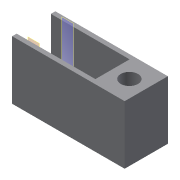
# Autodesk Inventor part: XRailVerticalExtension
Saved by Autodesk Inventor 2018 (Build 220112000, 112)
## iProperties
Created: 2019-02-14
Part Number: XRailVerticalExtension
Material: Generic
Document SubType Name: Modeling
Designer: ball
Density: 1 g/cm^3
Appearance: Default
Author: ball
Autodesk Inventor part; units mm, degrees
ref_plane "YZ Plane" through (0, 0, 0) normal (1, 0, 0) x (0, 1, 0)
ref_plane "XZ Plane" through (0, 0, 0) normal (0, 1, 0) x (-1, 0, 0)
ref_plane "XY Plane" through (0, 0, 0) normal (0, 0, 1) x (1, 0, 0)
ref_plane "Work Plane1" through (0, 0, 0) normal (0, 0, 1) x (1, 0, 0)
sketch "Sketch1" plane through (0, 0, 0) normal (0, 0, 1) x (1, 0, 0)
  line L0 (3, 16.51) -> (-3, 16.51) construction
  line L1 (-3, -16.51) -> (3, -16.51) construction
  line L2 (-9.525, -16.51) -> (-9.525, 173.99) construction
  line L3 (9.525, -16.51) -> (9.525, 173.99) construction
  line L4 (-9.525, -16.51) -> (53.975, -16.51)
  line L5 (53.975, -16.51) -> (53.975, 16.51)
  line L6 (53.975, 16.51) -> (-9.525, 16.51)
  line L7 (-9.525, 16.51) -> (-9.525, -16.51)
  point P0 (0, 0)
  dimension "d0" = 63.5
  constraints: 8 end point, 2 parallel, 1 horizontal, 1 perpendicular
  measures "d0" distance of L6.end L5.end
extrude "Extrusion1" add sketch "Sketch1" along normal blind 2.54
ref_plane "Work Plane2" through (0, 0, -19.304) normal (0, 0, -1) x (1, 0, 0)
sketch "Sketch2" plane through (0, 0, -19.304) normal (0, 0, -1) x (1, 0, 0)
  line L0 (-9.525, 16.51) -> (53.975, 16.51) projected
  line L1 (53.975, -16.51) -> (-9.525, -16.51) projected
  line L2 (-9.525, 16.51) -> (53.975, 16.51)
  line L3 (53.975, 16.51) -> (53.975, -16.51)
  line L4 (53.975, -16.51) -> (-9.525, -16.51)
  line L5 (-9.525, -16.51) -> (-9.525, 16.51)
  point P0 (0, 0)
  dimension "d3" = 63.5
  constraints: 8 end point, 2 parallel, 1 horizontal, 1 perpendicular
  measures "d3" distance of L1.start L4.end
extrude "Extrusion2" add sketch "Sketch2" along normal blind 2.54
sketch "Sketch3" plane through (-9.525, -16.51, 0) normal (0, -1, 0) x (1, 0, 0)
  line L0 (63.5, 0) -> (0, 0) projected
  line L1 (0, -19.304) -> (63.5, -19.304) projected
  line L2 (63.5, 0) -> (44.45, 0)
  line L3 (44.45, 0) -> (44.45, -19.304)
  line L4 (44.45, -19.304) -> (63.5, -19.304)
  line L5 (63.5, -19.304) -> (63.5, 0)
  point P0 (9.525, 0)
  dimension "d6" = 19.05
  constraints: 8 end point, 2 parallel, 1 horizontal, 1 perpendicular, 1 point on line
  measures "d6" distance of L4.end L3.end
extrude "Extrusion3" add sketch "Sketch3" against normal blind 33.02
sketch "Sketch4" plane through (-9.525, -16.51, 2.54) normal (0, -1, 0) x (1, 0, 0)
  line L0 (44.45, -21.844) -> (44.45, -2.54) construction
  line L1 (44.45, -12.192) -> (63.5, -12.192) construction
  point P0 (9.525, -2.54)
  point P1 (53.975, -12.192)
  constraints: 2 end point, 2 midpoint, 1 horizontal
hole "Hole1" at (44.45, -16.51, -9.652) direction (0, 1, 0) diameter 9.779 end through all
body "Solid1"
